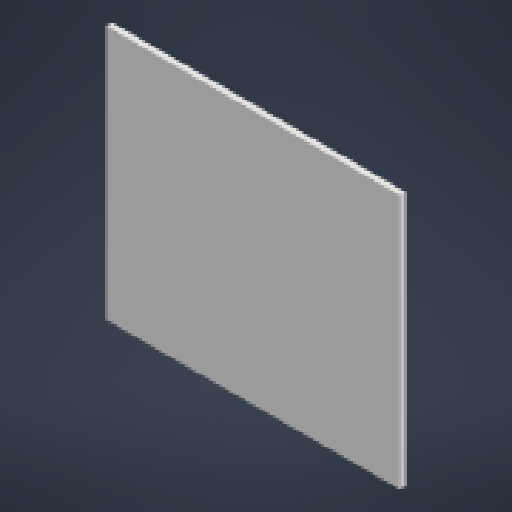
# Autodesk Inventor part: xpanel
Saved by Autodesk Inventor 2025.1 (Build 291241020, 241B)
## iProperties
Created: 2024-09-23
Part Number: xpanel
Material: Generic
Document SubType Name: Modeling
Designer: techn
Density: 1 g/cm^3
Appearance: Default
Author: techn
Autodesk Inventor part; units mm, degrees
ref_plane "YZ Plane" through (0, 0, 0) normal (1, 0, 0) x (0, 1, 0)
ref_plane "XZ Plane" through (0, 0, 0) normal (0, 1, 0) x (-1, 0, 0)
ref_plane "XY Plane" through (0, 0, 0) normal (0, 0, 1) x (1, 0, 0)
sketch "Sketch1" plane through (0, 0, 0) normal (0, 0, 1) x (1, 0, 0)
  line L0 (-18, -6) -> (162, -6) projected
  line L1 (162, 0) -> (162, -6) projected
  line L2 (-18, 0) -> (162, 0) projected
  line L3 (-18, -6) -> (-18, 0) projected
  line L4 (-4, 0) -> (2, 0) projected
  line L5 (2, 0) -> (2, 120) projected
  line L6 (-4, 120) -> (2, 120) projected
  line L7 (-4, 0) -> (-4, 120) projected
  line L8 (148, 0) -> (142, 0) projected
  line L9 (142, 0) -> (142, 120) projected
  line L10 (148, 120) -> (142, 120) projected
  line L11 (148, 0) -> (148, 120) projected
  line L12 (-18, 120) -> (162, 120) projected
  line L13 (162, 126) -> (162, 120) projected
  line L14 (-18, 126) -> (162, 126) projected
  line L15 (-18, 120) -> (-18, 126) projected
  line L16 (-4, -6) -> (148, -6)
  line L17 (148, -6) -> (148, 126)
  line L18 (148, 126) -> (-4, 126)
  line L19 (-4, 126) -> (-4, -6)
  line L20 (147, 125) -> (147, -5)
  line L21 (147, -5) -> (-3, -5)
  line L22 (-3, -5) -> (-3, 125)
  line L23 (-3, 125) -> (147, 125)
  point P0 (0, 0)
  dimension "d0" = 1
  constraints: 16 end point, 4 parallel, 2 perpendicular, 2 point on line, 1 horizontal, 3 other
  measures "d0" distance between parallel lines of L17 L20
extrude "Extrusion1" add sketch "Sketch1" along normal blind 3 contours L22 L6 L5 L2 | L2 L20 L21 L22 | L2 L9 L10 L20 | L5 L12 L9 L2 | L22 L23 L20 L10 L12 L6
body "Solid1"
